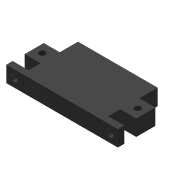
# Autodesk Inventor part: 00_laserdriver_Pcb
Saved by Autodesk Inventor 2019.4 (Build 234330000, 330)
## iProperties
Created: 2020-06-15
Part Number: 00_laserdriver_Pcb
Material: Generic
Document SubType Name: Modeling
Designer: diederichbenedict
Density: 1 g/cm^3
Appearance: Dark Gray
Author: diederichbenedict
Autodesk Inventor part; units mm, degrees
ref_plane "YZ Plane" through (0, 0, 0) normal (1, 0, 0) x (0, 1, 0)
ref_plane "XZ Plane" through (0, 0, 0) normal (0, 1, 0) x (-1, 0, 0)
ref_plane "XY Plane" through (0, 0, 0) normal (0, 0, 1) x (1, 0, 0)
sketch "Sketch1" plane through (0, 0, 0) normal (0, 1, 0) x (-1, 0, 0)
  line L0 (0, 0) -> (-50, 0)
  line L1 (-50, 0) -> (-50, 35)
  line L2 (-50, 35) -> (0, 35)
  line L3 (0, 35) -> (0, 0)
  line L4 (0, 23.5) -> (10, 23.5)
  line L5 (10, 23.5) -> (10, 11.5)
  line L6 (10, 11.5) -> (0, 11.5)
  line L7 (0, 11.5) -> (0, 23.5)
  line L8 (-50, 23.5) -> (-60, 23.5)
  line L9 (-60, 23.5) -> (-60, 11.5)
  line L10 (-60, 11.5) -> (-50, 11.5)
  line L11 (-50, 11.5) -> (-50, 23.5)
  circle A0 centre (5, 17.5) radius 2
  circle A1 centre (-55, 17.5) radius 2
  dimension "d0" = 50
  dimension "d1" = 35
  dimension "d2" = 10
  dimension "d3" = 12
  dimension "d4" = 11.5
  dimension "d5" = 10
  dimension "d6" = 4
  dimension "d7" = 4
  constraints: 24 end point, 6 parallel, 3 horizontal, 3 perpendicular, 2 centre point, 2 point on line
  measures "d0" distance of L1.end L2.end
  measures "d1" distance of L0.end L1.end
  measures "d2" distance of L5.end L6.end
  measures "d3" distance of L4.end L5.end
  measures "d4" distance between parallel lines of L4 L2
  measures "d5" distance of L10.end L9.end
  measures "d6" diameter of A0
  measures "d7" diameter of A1
extrude "Extrusion1" add sketch "Sketch1" along normal blind 10
sketch "Sketch2" plane through (0, 0, 35) normal (0, 0, 1) x (1, 0, 0)
  line L0 (50, 0) -> (0, 0) projected
  line L1 (50, 0) -> (50, 10) projected
  line L2 (0, 10) -> (50, 10) projected
  line L3 (0, 0) -> (0, 10) projected
  line L4 (0, 0) -> (-10, 0) projected
  line L5 (0, 0) -> (0, 10) projected
  line L6 (-10, 10) -> (0, 10) projected
  line L7 (-10, 0) -> (-10, 10) projected
  line L8 (50, 0) -> (60, 0) projected
  line L9 (60, 0) -> (60, 10) projected
  line L10 (50, 10) -> (60, 10) projected
  line L11 (50, 0) -> (50, 10) projected
  circle A0 centre (-5, 5) radius 2
  circle A1 centre (55, 5) radius 2
  dimension "d10" = 4
  dimension "d11" = 4
  constraints: 2 centre point
  measures "d10" diameter of A0
  measures "d11" diameter of A1
extrude "Extrusion2" add sketch "Sketch2" against normal blind 4
body "Solid1"
